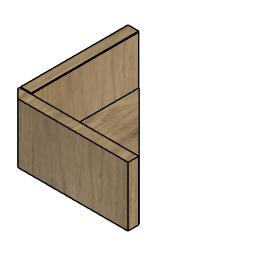
stretcher-brace (Autodesk Fusion 360 design; units mm, degrees)
Autodesk Fusion 360 part; units mm, degrees
sketch "Sketch1" plane through (0, 0, 0) normal (0, 0, 1) x (1, 0, 0)
  line L0 (0, 0) -> (203.2, 0)
  line L1 (203.2, 0) -> (203.2, 203.2) construction
  line L2 (203.2, 203.2) -> (0, 203.2) construction
  line L3 (0, 203.2) -> (0, 0)
  line L4 (203.2, 203.2) -> (19.05, 203.2) construction
  line L5 (19.05, 203.2) -> (19.05, 19.05)
  line L6 (19.05, 19.05) -> (203.2, 19.05)
  line L7 (203.2, 19.05) -> (203.2, 203.2) construction
  line L8 (0, 203.2) -> (19.05, 203.2)
  line L9 (203.2, 19.05) -> (203.2, 0)
  line L10 (19.05, 19.05) -> (0, 19.05)
  line L11 (19.05, 203.2) -> (203.2, 19.05)
  dimension "d1" = 203.2
  dimension "d3" = 203.2
  dimension "d4" = 184.15
  dimension "d5" = 184.15
  constraint horizontal L0
  constraint vertical L1
  constraint horizontal L2
  constraint vertical L3
  constraint coincident L0.start L3.end
  constraint horizontal L4
  constraint vertical L5
  constraint horizontal L6
  constraint vertical L7
  constraint coincident L3 L10.end
  constraint perpendicular L3 L10
  measures "d1" distance of L0.start L0.end
  measures "d3" distance of L0 L2
  measures "d4" distance of L1.end L4.end
  measures "d5" distance of L1.end L6.end
extrude "Extrude1" add sketch "Sketch1" along normal blind 19.05 contours L5 L6 L11 makes body 1 in component "Bottom"
chamfer "Chamfer1" distance 0.762 angle 45 2 faces at (141.8167, 19.05, 6.35) (19.05, 80.4333, 12.7) on bodies 1 in component "Bottom"
extrude "Extrude1'" add sketch "Sketch1" along normal blind 101.6 separate body contours L3 L5 L8 L10 makes body 2 in component "Side 1"
chamfer "Chamfer1'" distance 0.762 angle 45 2 faces at (19.05, 141.8167, 33.8667) (12.7, 19.05, 33.8667) on bodies 2 in component "Side 1"
extrude "Extrude1''" add sketch "Sketch1" along normal blind 101.6 separate body contours L0 L3 L6 L9 L10 makes body 3 in component "Side 2"
chamfer "Chamfer2" distance 0.762 angle 45 2 faces at (12.7, 19.05, 33.8667) (80.4333, 19.05, 33.8667) on bodies 3 in component "Side 2"
chamfer "Chamfer1''" distance 15.24 angle 45 1 edges at (0, 0, 50.8) on bodies 3 in component "Side 2"
component "Bottom" placed x (1, 0, 0) y (0, 1, 0) z (0, 0, 1) at (0, 0, 0)
component "Side 1" placed x (1, 0, 0) y (0, 1, 0) z (0, 0, 1) at (0, 0, 0)
component "Side 2" placed x (1, 0, 0) y (0, 1, 0) z (0, 0, 1) at (0, 0, 0)
equation "d3 = d1"
equation "d4 = d1 - 0.75 in"
equation "d5 = d4"
